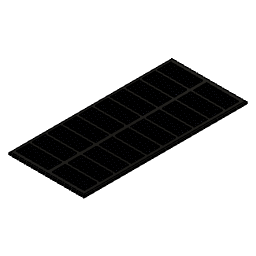
1W _5V (Autodesk Fusion 360 design; units mm, degrees)
Autodesk Fusion 360 part; units mm, degrees
sketch "Sketch1" plane through (0, 0, 0) normal (0, 0, 1) x (1, 0, 0)
  line L0 (34.5, 75) -> (-34.5, 75)
  line L1 (-34.5, 75) -> (-34.5, -75)
  line L2 (-34.5, -75) -> (34.5, -75)
  line L3 (34.5, -75) -> (34.5, 75)
  line L4 (34.5, 75) -> (-34.5, -75) construction
  line L5 (-34.5, 75) -> (34.5, -75) construction
  dimension "d1" = 69
  dimension "d2" = 150
  constraint horizontal L0
  constraint perpendicular L0 L1
  constraint parallel L0 L2
  constraint parallel L1 L3
  constraint coincident L4 origin
  constraint coincident L5 origin
  measures "d1" distance of L1.end L2.end
  measures "d2" distance of L0.end L1.end
extrude "Extrude1" add sketch "Sketch1" along normal blind 2
sketch "Sketch2" plane through (0, 0, 2) normal (0, 0, 1) x (-1, 0, 0)
  line L0 (-34.5, 75) -> (-34.5, -75)
  line L1 (-34.5, -75) -> (34.5, -75)
  line L2 (34.5, -75) -> (34.5, 75)
  line L3 (34.5, 75) -> (-34.5, 75)
  line L4 (2.25, 59) -> (31.75, 59)
  line L5 (31.75, 59) -> (31.75, 71)
  line L6 (31.75, 71) -> (2.25, 71)
  line L7 (2.25, 71) -> (2.25, 59)
  line L8 (2.25, 59) -> (31.75, 71) construction
  line L9 (31.75, 59) -> (2.25, 71) construction
  point P0 (17, 65)
  dimension "d5" = 29.5
  dimension "d6" = 12
  dimension "d7" = 10
  dimension "d8" = 17.5
  constraint horizontal L4
  constraint perpendicular L4 L5
  constraint parallel L4 L6
  constraint parallel L5 L7
  constraint coincident L8 P0
  constraint coincident L9 P0
  measures "d5" distance of L5.end L6.end
  measures "d6" distance of L4.end L5.end
  measures "d7" distance of L3 P0
  measures "d8" distance of L2 P0
extrude "Extrude2" add sketch "Sketch2" along normal blind 0.005 contours L4 L5 L6 L7
sketch "Sketch3" plane through (0, 0, 2.005) normal (0, 0, 1) x (-1, 0, 0)
  line L0 (2.25, 71) -> (2.25, 59)
  line L1 (2.25, 59) -> (31.75, 59)
  line L2 (31.75, 59) -> (31.75, 71)
  line L3 (31.75, 71) -> (2.25, 71)
  line L4 (31.75, 70.25) -> (2.25, 70.25)
  line L5 (2.25, 70.25) -> (2.25, 70)
  line L6 (2.25, 70) -> (31.75, 70)
  line L7 (31.75, 70) -> (31.75, 70.25)
  dimension "d11" = 0.25
  dimension "d12" = 0.75
  constraint horizontal L4
  constraint vertical L5
  constraint horizontal L6
  constraint vertical L7
  constraint coincident L2 L4.start
  measures "d11" distance of L4.start L6.end
  measures "d12" distance of L3 L4
extrude "Extrude3" add sketch "Sketch3" along normal blind 0.005 contours L0 L2 L4 L5 L6 L7
pattern_linear "R-Pattern1" count 8 spacing 1.475 along (0, 1, 0) of "Extrude3"
pattern_linear "R-Pattern2" count 10 spacing 14.45 along (0, 1, 0) count 2 spacing 33 along (1, 0, 0) of "Extrude2", "Extrude3", "R-Pattern1"
fillet "Fillet1" radius 0.75 4 edges at (0, -75, 2) (34.5, 0, 2) (-34.5, 0, 2) (0, 75, 2)
sketch "Sketch4" plane through (0, 0, 0) normal (0, 0, -1) x (1, 0, 0)
  line L0 (34.5, -75) -> (34.5, 75)
  line L1 (34.5, 75) -> (-34.5, 75)
  line L2 (-34.5, 75) -> (-34.5, -75)
  line L3 (-34.5, -75) -> (34.5, -75)
  line L4 (-8.5, -67) -> (-12.5, -67)
  line L5 (-12.5, -67) -> (-12.5, -71)
  line L6 (-12.5, -71) -> (-8.5, -71)
  line L7 (-8.5, -71) -> (-8.5, -67)
  line L8 (-8.5, -67) -> (-12.5, -71) construction
  line L9 (-12.5, -67) -> (-8.5, -71) construction
  line L10 (12.5, -67) -> (8.5, -67)
  line L11 (8.5, -67) -> (8.5, -71)
  line L12 (8.5, -71) -> (12.5, -71)
  line L13 (12.5, -71) -> (12.5, -67)
  line L14 (12.5, -67) -> (8.5, -71) construction
  line L15 (8.5, -67) -> (12.5, -71) construction
  circle A0 centre (-17.5, -68.5) radius 2.25
  circle A1 centre (-17.5, -68.5) radius 2.625
  circle A2 centre (-17.5, -68.5) radius 1.75
  line L16 (-17.75, -66.7679) -> (-17.75, -70.2321)
  line L17 (-17.25, -70.2321) -> (-17.25, -66.7679)
  circle A3 centre (17.5, -68.5) radius 2.625
  circle A4 centre (17.5, -68.5) radius 2.25
  circle A5 centre (17.5, -68.5) radius 1.75
  line L18 (17.25, -66.7679) -> (17.25, -70.2321)
  line L19 (17.75, -70.2321) -> (17.75, -66.7679)
  line L20 (15.7679, -68.75) -> (19.2321, -68.75)
  line L21 (15.7679, -68.25) -> (19.2321, -68.25)
  circle A6 centre (0, -72.5) radius 2
  line L22 (-8.5, 2.0004) -> (-12.5, 2.0004)
  line L23 (-12.5, 2.0004) -> (-12.5, -1.9996)
  line L24 (-12.5, -1.9996) -> (-8.5, -1.9996)
  line L25 (-8.5, -1.9996) -> (-8.5, 2.0004)
  line L26 (-8.5, 2.0004) -> (-12.5, -1.9996) construction
  line L27 (-12.5, 2.0004) -> (-8.5, -1.9996) construction
  line L28 (12.5, 2.0004) -> (8.5, 2.0004)
  line L29 (8.5, 2.0004) -> (8.5, -1.9996)
  line L30 (8.5, -1.9996) -> (12.5, -1.9996)
  line L31 (12.5, -1.9996) -> (12.5, 2.0004)
  line L32 (12.5, 2.0004) -> (8.5, -1.9996) construction
  line L33 (8.5, 2.0004) -> (12.5, -1.9996) construction
  line L34 (4.75, 16.5) -> (-4.75, 16.5)
  line L35 (-4.75, 16.5) -> (-4.75, -16.5)
  line L36 (-4.75, -16.5) -> (4.75, -16.5)
  line L37 (4.75, -16.5) -> (4.75, 16.5)
  line L38 (4.75, 16.5) -> (-4.75, -16.5) construction
  line L39 (-4.75, 16.5) -> (4.75, -16.5) construction
  line L40 (-10.5, -69) -> (-10.5, 0.0004)
  line L41 (10.5, 0.0004) -> (10.5, -69)
  point P0 (-10.5, -69)
  point P1 (10.5, -69)
  point P2 (-10.5, 0.0004)
  point P3 (10.5, 0.0004)
  dimension "d25" = 4
  dimension "d26" = 4
  dimension "d27" = 4
  dimension "d28" = 4
  dimension "d29" = 4
  dimension "d30" = 22
  dimension "d31" = 4
  dimension "d32" = 22
  dimension "d33" = 4.5
  dimension "d34" = 5.25
  dimension "d35" = 3.5
  dimension "d36" = 0.25
  dimension "d37" = 0.25
  dimension "d38" = 17
  dimension "d39" = 6.5
  dimension "d40" = 5.25
  dimension "d41" = 6.5
  dimension "d42" = 17
  dimension "d43" = 4.5
  dimension "d44" = 3.5
  dimension "d45" = 0.25
  dimension "d46" = 0.25
  dimension "d47" = 0.25
  dimension "d48" = 0.25
  dimension "d49" = 4
  dimension "d50" = 2.5
  dimension "d51" = 4
  dimension "d52" = 4
  dimension "d53" = 4
  dimension "d54" = 4
  dimension "d55" = 9.5
  dimension "d56" = 33
  constraint horizontal L4
  constraint perpendicular L4 L5
  constraint parallel L4 L6
  constraint parallel L5 L7
  constraint coincident L8 P0
  constraint coincident L9 P0
  constraint horizontal L10
  constraint perpendicular L10 L11
  constraint parallel L10 L12
  constraint parallel L11 L13
  constraint coincident L14 P1
  constraint coincident L15 P1
  constraint concentric A0 A1
  constraint concentric A0 A2
  constraint coincident A2 L16.start
  constraint coincident A2 L16.end
  constraint vertical L16
  constraint coincident A2 L17.start
  constraint coincident A2 L17.end
  constraint parallel L16 L17
  constraint concentric A3 A4
  constraint concentric A4 A5
  constraint coincident A5 L18.start
  constraint coincident A5 L18.end
  constraint vertical L18
  constraint coincident A5 L19.start
  constraint coincident A5 L19.end
  constraint parallel L18 L19
  constraint coincident A5 L20.start
  constraint coincident A5 L20.end
  constraint perpendicular L18 L20
  constraint coincident A5 L21.start
  constraint coincident A5 L21.end
  constraint perpendicular L18 L21
  constraint horizontal L22
  constraint perpendicular L22 L23
  constraint parallel L22 L24
  constraint parallel L23 L25
  constraint coincident L26 P2
  constraint coincident L27 P2
  constraint horizontal L28
  constraint perpendicular L28 L29
  constraint parallel L28 L30
  constraint parallel L29 L31
  constraint coincident L32 P3
  constraint coincident L33 P3
  constraint horizontal L34
  constraint perpendicular L34 L35
  constraint parallel L34 L36
  constraint parallel L35 L37
  constraint coincident L38 origin
  constraint coincident L39 origin
  constraint coincident P0 L40.start
  constraint coincident P2 L40.end
  constraint parallel L0 L40
  constraint coincident P3 L41.start
  constraint coincident P1 L41.end
  constraint parallel L0 L41
  measures "d25" distance of L5.end L6.end
  measures "d26" distance of L4.end L5.end
  measures "d27" distance of L11.end L12.end
  measures "d28" distance of L10.end L11.end
  measures "d29" distance of L3 L6
  measures "d30" distance of L2 L5
  measures "d31" distance of L3 L12
  measures "d32" distance of L0 L13
  measures "d33" diameter of A0
  measures "d34" diameter of A1
  measures "d35" diameter of A2
  measures "d36" distance of A0.centre L16
  measures "d37" distance of A0.centre L17
  measures "d38" distance of L2 A0.centre
  measures "d39" distance of L3 A0.centre
  measures "d40" diameter of A3
  measures "d41" distance of L3 A3.centre
  measures "d42" distance of L0 A3.centre
  measures "d43" diameter of A4
  measures "d44" diameter of A5
  measures "d45" distance of A3.centre L18
  measures "d46" distance of A3.centre L19
  measures "d47" distance of A3.centre L20
  measures "d48" distance of A3.centre L21
  measures "d49" diameter of A6
  measures "d50" distance of L3 A6.centre
  measures "d51" distance of L23.end L24.end
  measures "d52" distance of L22.end L23.end
  measures "d53" distance of L29.end L30.end
  measures "d54" distance of L28.end L29.end
  measures "d55" distance of L35.end L36.end
  measures "d56" distance of L34.end L35.end
extrude "Extrude4" add sketch "Sketch4" along normal blind 0.01 contours L4 L5 L6 L7 | L10 L11 L12 L13 | A0 | A2 L16 L17 | A4 | A5 L19 L20 L21 | A5 L18 L19 L21 | L18 L19 L20 L21 | A5 L18 L19 L20 | A5 L18 L20 L21
extrude "Extrude5" add sketch "Sketch4" along normal blind 0.005 contours A1 | A2 L17 | A2 L16 | A3 | A5 L19 L21 | A5 L19 L20 | A5 L18 L21 | A5 L18 L20
extrude "Extrude6" add sketch "Sketch4" along normal blind 0.25 contours A6
fillet "Fillet2" radius 2 1 edges at (-1.8647, 73.2232, -0.25)
mirror "Mirror1" about plane through (0, 0, 0) normal (0, 1, 0) of "Extrude4", "Extrude5", "Extrude6", "Fillet2"
extrude "Extrude7" add sketch "Sketch4" along normal blind 0.005 contours L34 L35 L36 L37
sketch "Sketch5" plane through (0, 0, -0.005) normal (0, 0, -1) x (1, 0, 0)
  line L0 (4.75, -16.5) -> (4.75, 16.5)
  line L1 (4.75, 16.5) -> (-4.75, 16.5)
  line L2 (-4.75, 16.5) -> (-4.75, -16.5)
  line L3 (-4.75, -16.5) -> (4.75, -16.5)
  line L4 (3.1687, -14.7152) -> (3.1687, 14.8365) construction
  line L5 (3.1687, 14.8365) -> (-3.0949, 14.8365) construction
  line L6 (-3.0949, 14.8365) -> (-3.0949, -14.7152) construction
  line L7 (-3.0949, -14.7152) -> (3.1687, -14.7152) construction
  dimension "d69" = 5
  text T0 "150X69" font "Verdana" height 5 align centre middle in box 29.5517 x 6.2636 at (3.1687, -14.7152) x (0, 1) y (-1, 0) spacing 1
extrude "Extrude8" add sketch "Sketch4" along normal blind 0.005 contours L22 L23 L24 L25 | L28 L29 L30 L31
extrude "Extrude9" add sketch "Sketch5" along normal blind 0.005 text T0
equation "d31 = d25"
equation "d32 = d30"
equation "d37 = d36"
equation "d46 = d45"
equation "d47 = d45"
equation "d48 = d47"
